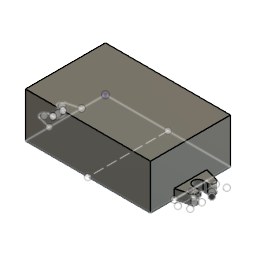
mid360_dcdc_v0_1 (Autodesk Fusion 360 design; units mm, degrees)
part number: 2026-05-28-15-28-27-091
Autodesk Fusion 360 part; units mm, degrees
sketch "草图1" plane through (0, 0, 0) normal (0, 1, 0) x (1, 0, 0)
  line L0 (0, 0) -> (50, 0)
  line L1 (50, 0) -> (50, -32)
  line L2 (50, -32) -> (0, -32)
  line L3 (0, -32) -> (0, 0)
  line L4 (50, -16) -> (51, -16) construction
  line L5 (51, -16) -> (53, -16) construction
  line L6 (53, -8.9008) -> (53, -24.056) construction
  line L7 (53, -14) -> (54.8904, -14)
  line L8 (56.4575, -7.9511) -> (56.4575, -22.5669) construction
  line L9 (50, -9.5) -> (50, -22.5)
  line L10 (50, -9.5) -> (55.296, -10.9191)
  arc A0 (54.8904, -14) -> (55.296, -10.9191) centre (54.8904, -12.4328) ccw
  line L11 (50, -22.5) -> (55.296, -21.0809)
  arc A1 (55.296, -21.0809) -> (54.8904, -18) centre (54.8904, -19.5672) ccw
  line L12 (53, -18) -> (54.8904, -18)
  line L13 (53, -18) -> (54.8904, -18)
  line L14 (56.4575, -18) -> (56.5, -18)
  arc A2 (53, -14) -> (53, -18) centre (53, -16) ccw
  line L15 (25, 0) -> (25, -32) construction
  line L16 (25, 0) -> (25, -32) construction
  line L17 (0, -9.5) -> (-5.296, -10.9191)
  arc A3 (-5.296, -10.9191) -> (-4.8904, -14) centre (-4.8904, -12.4328) ccw
  line L18 (-3, -14) -> (-4.8904, -14)
  arc A4 (-3, -18) -> (-3, -14) centre (-3, -16) ccw
  line L19 (-3, -18) -> (-4.8904, -18)
  arc A5 (-4.8904, -18) -> (-5.296, -21.0809) centre (-4.8904, -19.5672) ccw
  line L20 (0, -22.5) -> (-5.296, -21.0809)
  point P0 (50, -16)
  point P1 (56.5, -14)
  dimension "d1" = 50
  dimension "d2" = 32
  dimension "d3" = 1
  dimension "d4" = 2
  dimension "d5" = 3.5
  dimension "d6" = 13
  dimension "d7" = 75
  dimension "d8" = 1.5672
  constraint horizontal L0
  constraint vertical L1
  constraint horizontal L2
  constraint vertical L3
  constraint coincident L0.start L3.end
  constraint midpoint L1 P0
  constraint coincident P0 L4.start
  constraint perpendicular L1 L4
  constraint perpendicular L1 L5
  constraint coincident L5.end A2.centre
  constraint coincident L4.end A2
  constraint perpendicular L5 L6
  constraint coincident L6 L7.start
  constraint coincident L6 L12.start
  constraint coincident L5.end L6
  constraint coincident L7.start A2.start
  constraint tangent L7 A2
  constraint perpendicular L6 L7
  constraint coincident L12.start L13.start
  constraint tangent L13 A2
  constraint perpendicular L6 L13
  constraint perpendicular L8 L14
  constraint coincident L1 L9.start
  constraint coincident L1 L9.end
  constraint symmetric L5 L9.start L9.end
  constraint coincident P1 L7
  constraint tangent L7 A0
  constraint tangent L10 A0
  constraint tangent L8 A0
  constraint symmetric L5 L7.start L12.start
  constraint symmetric L5 L7.end A1.end
  constraint symmetric L5 L10.end L11.end
  constraint symmetric L5 A0 A1
  constraint coincident L8 L14.start
  constraint collinear L13 L14
  constraint midpoint L0 L15.start
  constraint midpoint L2 L15.end
  constraint symmetric L7.start L15 L18.start
  constraint symmetric L12.start L15 A4.start
  constraint symmetric L9.start L15 L17.start
  constraint symmetric L7.end L15 A3.end
  constraint symmetric L10.end L15 L17.end
  constraint symmetric A0 L15 A3
  constraint symmetric L9.end L15 L20.start
  constraint symmetric L11.end L15 A5.end
  constraint symmetric A1.end L15 L19.end
  constraint symmetric A1 L15 A5
  constraint symmetric A2 L15 A4
  constraint symmetric L16.start L15 L15.start
  constraint symmetric L16.end L15 L15.end
  measures "d1" distance of L0.start L0.end
  measures "d2" distance of L0.start L2.end
  measures "d3" distance of P0 L4.end
  measures "d4" distance of L4.end L5.end
  measures "d5" distance of L7.start P1
  measures "d6" distance of L9.start L9.end
  measures "d7" angle of L9 L10
  measures "d8" radius of A0
extrude "拉伸1" add sketch "草图1" along normal blind 18 contours L0 L1 L2 L3 L9
extrude "拉伸2" add sketch "草图1" along normal blind 3.8 contours L3 L17 A3 L18 A4 L19 A5 L20 | L1 L7 L9 L10 A0 L11 A1 L12 L13 A2
